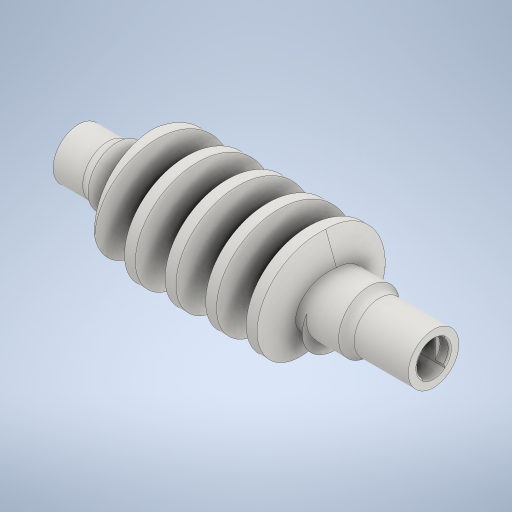
# Autodesk Inventor part: Tornillo helicoidal
Saved by Autodesk Inventor 2023 (Build 270158000, 158)
## iProperties
Created: 2022-12-03
Part Number: Tornillo helicoidal
Material: Steel, Mild
Document SubType Name: Modeling
Designer: sergi
Categories: <?xml version="1.0" encoding="UTF-16"?> <MemberInstance><Categories><FamilyTemplate><FamilyTemplateParameter ValueType="xs:double" Id="1" ObjectReferenceKey="da_z" ObjectType="kUserParameterObject"/><FamilyTemplateParameter ValueType="xs:double" Id="2" ObjectReferenceKey="da_b" ObjectType="kUserParameterObject"/><FamilyTemplateParameter ValueType="xs:double" Id="3" ObjectReferenceKey="da_beta" ObjectType="kUserParameterObject"/><FamilyTemplateParameter ValueType="xs:double" Id="4" ObjectReferenceKey="da_m" ObjectType="kUserParameterObject"/><FamilyTemplateParameter ValueType="xs:double" Id="5" ObjectReferenceKey="da_alpha" ObjectType="kUserParameterObject"/><FamilyTemplateParameter ValueType="xs:double" Id="6" ObjectReferenceKey="da_da" ObjectType="kUserParameterObject"/><FamilyTemplateParameter ValueType="xs:double" Id="7" ObjectReferenceKey="da_aw" ObjectType="kUserParameterObject"/><FamilyTemplateParameter ValueType="xs:double" Id="8" ObjectReferenceKey="da_px" ObjectType="kUserParameterObject"/><FamilyTemplateParameter ValueType="xs:double" Id="9" ObjectReferenceKey="da_d" ObjectType="kUserParameterObject"/><FamilyTemplateParameter ValueType="xs:string" Id="10" ObjectReferenceKey="EAIAABAAAADKGAAAAAAAAIAAAAAAAAAA" ObjectType="83910656" SubObjectId="SurfaceGeometry"/></FamilyTemplate><ParamToTemplateMap><ParamToTemplate CategoryParameter="//CategoryParameter[@InternalName='046C89C9-8512-4d59-83FE-43B91F4F132A']" TemplateParameter="1"/><ParamToTemplate CategoryParameter="//CategoryParameter[@InternalName='2552DF32-E462-4b46-AEBF-C6C7768E72AC']" TemplateParameter="2"/><ParamToTemplate CategoryParameter="//CategoryParameter[@InternalName='C9EE641D-15FC-4fae-A226-E94C4372FDD7']" TemplateParameter="3"/><ParamToTemplate><ParamToTemplate CategoryParameter="//CategoryParameter[@InternalName='00B6519A-459B-49c7-AD84-2E56D39A5744']" ConstantValue="0.000000"/></ParamToTemplate><ParamToTemplate><ParamToTemplate CategoryParameter="//CategoryParameter[@InternalName='04B31F0E-C7A6-4894-AA32-9629BEFACF47']" ConstantValue="1.000000"/></ParamToTemplate><ParamToTemplate><ParamToTemplate CategoryParameter="//CategoryParameter[@InternalName='43CBEC2E-7847-49e7-A936-2F7889FCB2D9']" ConstantValue="0.200000"/></ParamToTemplate><ParamToTemplate><ParamToTemplate CategoryParameter="//CategoryParameter[@InternalName='B1EFC894-105D-4ebd-86BF-FA20ED196853']" ConstantValue="0.300000"/></ParamToTemplate><ParamToTemplate><ParamToTemplate CategoryParameter="//CategoryParameter[@InternalName='51175063-3D10-4879-93E8-6246FE8B403D']" ConstantValue="2067000000.000000"/></ParamToTemplate><ParamToTemplate><ParamToTemplate CategoryParameter="//CategoryParameter[@InternalName='A3A52E27-4454-46a9-B0BD-C932399B70AF']" ConstantValue="0.270000"/></ParamToTemplate><ParamToTemplate CategoryParameter="//CategoryParameter[@InternalName='91B76062-C214-41d9-B1B9-14D2AB99603D']" TemplateParameter="4"/><ParamToTemplate CategoryParameter="//CategoryParameter[@InternalName='2D373A89-B862-43d6-8D0B-0CBF12AB9F6C']" TemplateParameter="5"/><ParamToTemplate CategoryParameter="//CategoryParameter[@InternalName='37777632-D6A2-4fac-9D53-DB8ACD95C989']" TemplateParameter="6"/><ParamToTemplate CategoryParameter="//CategoryParameter[@InternalName='FD1017F1-B727-4f7e-9707-0F86F1FF9423']" TemplateParameter="7"/><ParamToTemplate CategoryParameter="//CategoryParameter[@InternalName='3BF567DA-17EF-48d8-80EA-D119B07F6463']" TemplateParameter="8"/><ParamToTemplate CategoryParameter="//CategoryParameter[@InternalName='BF5A1E7E-5373-4a22-AAD3-F583781FCF3C']" TemplateParameter="9"/><ParamToTemplate><ParamToTemplate CategoryParameter="//CategoryParameter[@InternalName='D4F72237-D604-435a-AD0B-F738B7463A00']" ConstantValue="1.000000"/></ParamToTemplate><ParamToTemplate CategoryParameter="//CategoryParameter[@InternalName='27C3BAF2-7550-4e4b-AE2C-0DB134B7D9B7']" TemplateParameter="10"/></ParamToTemplateMap><Category DisplayName="Gear" InternalName="DC85795E-93AB-48d5-8EEE-5A27447B64BD" Mnemonic="Gear"><CategoryParameter DisplayName="z" InternalName="046C89C9-8512-4d59-83FE-43B91F4F132A" Mnemonic="z"/><CategoryParameter DisplayName="b|.1|" InternalName="2552DF32-E462-4b46-AEBF-C6C7768E72AC" Mnemonic="b"/><CategoryParameter DisplayName="||g|" InternalName="C9EE641D-15FC-4fae-A226-E94C4372FDD7" Mnemonic="beta"/><CategoryParameter DisplayName="x" InternalName="00B6519A-459B-49c7-AD84-2E56D39A5744" Mnemonic="x"/><CategoryParameter DisplayName="a*" InternalName="04B31F0E-C7A6-4894-AA32-9629BEFACF47" Mnemonic="a"/><CategoryParameter DisplayName="c*" InternalName="43CBEC2E-7847-49e7-A936-2F7889FCB2D9" Mnemonic="c"/><CategoryParameter DisplayName="r|.f|*" InternalName="B1EFC894-105D-4ebd-86BF-FA20ED196853" Mnemonic="rf"/><CategoryParameter DisplayName="E" InternalName="51175063-3D10-4879-93E8-6246FE8B403D" Mnemonic="E"/><CategoryParameter DisplayName="||m|" InternalName="A3A52E27-4454-46a9-B0BD-C932399B70AF" Mnemonic="mi"/><Category DisplayName="WormGear" InternalName="1B25C7EF-093B-4025-B3D3-619CD2A4550C" Mnemonic="WormGear"><CategoryParameter DisplayName="m" InternalName="91B76062-C214-41d9-B1B9-14D2AB99603D" Mnemonic="m"/><CategoryParameter DisplayName="||a|" InternalName="2D373A89-B862-43d6-8D0B-0CBF12AB9F6C" Mnemonic="alpha"/><CategoryParameter DisplayName="d|.a|" InternalName="37777632-D6A2-4fac-9D53-DB8ACD95C989" Mnemonic="da"/><CategoryParameter DisplayName="a|.w|" InternalName="FD1017F1-B727-4f7e-9707-0F86F1FF9423" Mnemonic="aw"/><CategoryParameter DisplayName="p|.x|" InternalName="3BF567DA-17EF-48d8-80EA-D119B07F6463" Mnemonic="px"/><CategoryParameter DisplayName="d" InternalName="BF5A1E7E-5373-4a22-AAD3-F583781FCF3C" Mnemonic="d"/><CategoryParameter DisplayName="k|.mat|" InternalName="D4F72237-D604-435a-AD0B-F738B7463A00" Mnemonic="Coef"/><CategoryParameter DisplayName="PitchDiameter" InternalName="27C3BAF2-7550-4e4b-AE2C-0DB134B7D9B7" Mnemonic="IDS_PITCHDIAM"/></Category></Category></Categories></MemberInstance>
Density: 7.86 g/cm^3
Appearance: Steel
CustomPartVersion: 1
Author: sergi
Autodesk Inventor part; units mm, degrees
ref_plane "YZ Plane" through (0, 0, 0) normal (1, 0, 0) x (0, 1, 0)
ref_plane "XZ Plane" through (0, 0, 0) normal (0, 1, 0) x (-1, 0, 0)
ref_plane "XY Plane" through (0, 0, 0) normal (0, 0, 1) x (1, 0, 0)
sketch "Boceto de cuerpo base" plane through (0, 0, 0) normal (1, 0, 0) x (0, 1, 0)
  circle A0 centre (0, 0) radius 9.1
  dimension "d5" = 18.2
extrude "Cuerpo base" add sketch "Boceto de cuerpo base" along normal mid plane 30
sketch "Sketch5" plane through (15, 0, 0) normal (1, 0, 0) x (0, 0, -1)
  circle A0 centre (0, 0) radius 9.1 projected
  circle A1 centre (0, 0) radius 7.1
  dimension "d59" = 14.2
  constraints: 1 centre point, 1 coincident
  measures "d59" diameter of A1
surface extrude "Diámetro de separación" sketch "Sketch5" against normal through all shown no curves A1
chamfer "Chamfer1" distance 1.6015 distance2 4.4 1 edges at (15, -9.1, 0) measured on face at (14.5, -9.1, 0)
chamfer "Chamfer2" distance 1.6015 distance2 4.4 1 edges at (-15, -9.1, 0) measured on face at (-14.5, -9.1, 0)
sketch "Boceto de diente" plane through (0, 0, 0) normal (0, 0, 1) x (1, 0, 0)
  line L0 (0, 21.74) -> (0, 10.96) projected
  line L1 (-24.323, 9.191) -> (-22.6884, 4.7)
  line L2 (-21.2939, 4.7) -> (-19.6593, 9.191)
  line L3 (-50.5346, 0) -> (-37.4554, 0) projected
  line L4 (-24.323, 9.191) -> (-21.9911, 9.191)
  line L5 (-21.9911, 9.191) -> (-19.6593, 9.191)
  line L6 (-22.6884, 4.7) -> (-21.9911, 4.7)
  line L7 (-21.9911, 4.7) -> (-21.2939, 4.7)
  line L8 (-21.9911, 7.1) -> (-20.4204, 7.1) construction
  line L9 (-21.9911, 9.191) -> (-21.9911, 4.7) construction
  dimension "d24" = 110
  dimension "d25" = 21.9912
  dimension "d26" = 1.5708
  dimension "d27" = 4.7
  dimension "d28" = 7.1
  dimension "d29" = 9.191
  constraints: 16 end point, 3 equal length, 3 parallel, 2 collinear, 2 point on line
  measures "d24" angle of L6 L1
  measures "d25" distance from line of L0 L4.end
  measures "d26" distance of L8.start L8.end
  measures "d27" distance between parallel lines of L3 L6
  measures "d28" distance between parallel lines of L3 L8
  measures "d29" distance between parallel lines of L3 L4
feature "Diente" [suppressed]
pattern_circular "Patrón de diente" [suppressed]
coil "Diente izquierdo" sketch "Boceto de diente" operation cut axis through (-10, 0, 0) along (1, 0, 0) pitch 6.2832 turns 7 hand left
pattern_of_one "Patrón de diente izquierdo"
sketch "Boceto6" plane through (15, 0, 0) normal (1, 0, 0) x (0, 0, -1)
  circle A0 centre (0, 0) radius 4.7
  constraints: 1 centre point, 1 coincident
extrude "Extrusión2" add sketch "Boceto6" along normal blind 5
sketch "Boceto7" plane through (20, 0, 0) normal (1, 0, 0) x (0, 0, -1)
  circle A0 centre (0, 0) radius 3.9
  dimension "d83" = 7.8
  constraints: 1 centre point, 1 coincident
  measures "d83" diameter of A0
extrude "Extrusión3" add sketch "Boceto7" along normal blind 10
sketch "Boceto8" plane through (30, 0, 0) normal (1, 0, 0) x (0, 0, -1)
  line L0 (1.5, -2) -> (1.5, 2)
  line L1 (-1.5, 2) -> (-1.5, -2)
  line L2 (-1.5, -5) -> (1.5, 5) construction
  line L3 (1.5, -5) -> (-1.5, 5) construction
  arc A0 (1.5, 2) -> (-1.5, 2) centre (0, 0) ccw
  arc A1 (-1.5, -2) -> (1.5, -2) centre (0, 0) ccw
  line L4 (-1.75, -2.1213) -> (-1.75, 2.1213)
  arc A2 (1.75, 2.1213) -> (-1.75, 2.1213) centre (0, 0) ccw
  line L5 (1.75, 2.1213) -> (1.75, -2.1213)
  arc A3 (-1.75, -2.1213) -> (1.75, -2.1213) centre (0, 0) ccw
  dimension "d86" = 3
  dimension "d87" = 10
  dimension "d89" = 0.25
  constraints: 12 end point, 8 point on circle, 4 centre point, 2 midpoint, 2 parallel, 1 coincident, 3 other
  measures "d86" distance of L3.end L2.end
  measures "d87" distance of L2.end L3.start
  measures "d89" distance between parallel lines of L1 L4
extrude "Extrusión4" cut sketch "Boceto8" against normal blind 8 contours A1 L1 A0 L0 | L4 A2 L5 A3
sketch "Boceto9" plane through (30, 0, 0) normal (1, 0, 0) x (0, 0, -1)
  circle A0 centre (0, 0) radius 3.9 projected
  constraints: 1 coincident
hole "Agujero1" at (30, 0, 0) direction (-1, 0, 0) diameter 5 depth 1.5
fillet "Empalme1" radius 2 1 edges at (20, 0, 3.9)
fillet "Empalme2" radius 0.25 2 edges at (30, 0, -2.5) (30, 0, 2.5)
sketch "Boceto10" plane through (-15, 0, 0) normal (-1, 0, 0) x (0, 0, 1)
  circle A0 centre (0, 0) radius 3.9 projected
  circle A1 centre (0, 0) radius 4.5
  dimension "d101" = 9
  constraints: 1 centre point, 1 coincident
  measures "d101" diameter of A1
extrude "Extrusión5" add sketch "Boceto10" along normal blind 4 contours A0 | A1
sketch "Boceto11" plane through (-19, 0, 0) normal (-1, 0, 0) x (0, 0, 1)
  circle A0 centre (0, 0) radius 3.9
  dimension "d104" = 7.8
  constraints: 1 centre point, 1 coincident
  measures "d104" diameter of A0
extrude "Extrusión6" add sketch "Boceto11" along normal blind 6
fillet "Empalme3" radius 2 1 edges at (-19, 0, -3.9)
equation "\"d6\" = da_b"
equation "\"d8\" = fd_cham1"
equation "\"d9\" = 0.5 * fd_cham2"
equation "\"d10\" = fd_cham1"
equation "\"d11\" = 0.5 * fd_cham2"
equation "\"d25\" = fd_dist"
equation "\"d26\" = 0.25 * da_px"
equation "\"d27\" = 0.5 * da_df"
equation "\"d28\" = 0.5 * da_d"
equation "\"d29\" = 0.505 * da_da"
equation "\"d32\" = fd_n"
equation "\"da_rightdir\" = 0"
equation "\"d64\" = fd_n"
equation "\"d5\" = da_da"
equation "\"d59\" = da_d"
equation "\"da_aw\" = 27.78571"
equation "\"da_b\" = 30"
equation "\"da_df\" = 9.4"
equation "\"da_da\" = 18.2"
equation "\"fd_cham2\" = da_da - da_df"
equation "\"fd_cham1\" = 0.181985 * fd_cham2"
equation "\"da_d\" = 14.2"
equation "\"da_px\" = 6.283185"
equation "\"da_alfat\" = 20deg"
equation "\"d49\" = da_aw"
equation "\"d79\" = da_aw"
equation "\"fd_dist\" = 21.991149"
equation "\"fd_n\" = 7"
body "Solid1"
body "Srf1"
